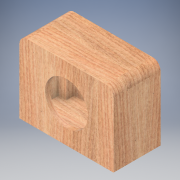
# Autodesk Inventor part: speakerBox
Saved by Autodesk Inventor 2017 (Build 210142000, 142)
## iProperties
Created: 2018-07-22
Part Number: speakerBox
Material: Wood (Birch)
Document SubType Name: Modeling
Designer: Jake
Density: 0.55 g/cm^3
Appearance: Birch - Natural Polished
Author: Jake
Autodesk Inventor part; units mm, degrees
ref_plane "YZ Plane" through (0, 0, 0) normal (1, 0, 0) x (0, 1, 0)
ref_plane "XZ Plane" through (0, 0, 0) normal (0, 1, 0) x (-1, 0, 0)
ref_plane "XY Plane" through (0, 0, 0) normal (0, 0, 1) x (1, 0, 0)
sketch "Sketch1" plane through (0, 0, 0) normal (0, 1, 0) x (-1, 0, 0)
  line L0 (152.4, 76.2) -> (-152.4, 76.2)
  line L1 (-152.4, 76.2) -> (-152.4, -76.2)
  line L2 (-152.4, -76.2) -> (152.4, -76.2)
  line L3 (152.4, -76.2) -> (152.4, 76.2)
  point P0 (0, 0)
  point P1 (152.4, 0)
  point P2 (0, -76.2)
  dimension "d0" = 152.4
  dimension "d1" = 304.8
  constraints: 8 end point, 2 midpoint, 2 parallel, 1 horizontal, 1 horizontal alignment, 1 perpendicular, 1 vertical alignment
  measures "d0" distance of L2.end L0.start
  measures "d1" distance of L1.end L2.end
extrude "Extrusion1" add sketch "Sketch1" along normal blind 15.875
sketch "Sketch4" plane through (0, 15.875, 0) normal (0, 1, 0) x (1, 0, 0)
  line L0 (-152.4, -76.2) -> (152.4, -76.2) projected
  line L1 (152.4, -76.2) -> (152.4, 76.2) projected
  line L2 (152.4, 76.2) -> (-152.4, 76.2) projected
  line L3 (-152.4, 76.2) -> (-152.4, -76.2) projected
  line L4 (-152.4, -76.2) -> (152.4, -76.2) projected
  line L5 (-152.4, -76.2) -> (136.525, -76.2)
  line L6 (136.525, -76.2) -> (136.525, -60.325)
  line L7 (136.525, -60.325) -> (-152.4, -60.325)
  line L8 (-152.4, -60.325) -> (-152.4, -76.2)
  point P0 (0, 0)
  dimension "d4" = 15.875
  dimension "d5" = 15.875
  constraints: 8 end point, 2 parallel, 1 horizontal, 1 perpendicular
  measures "d4" distance between parallel lines of L0 L7
  measures "d5" distance between parallel lines of L1 L6
extrude "Extrusion2" add sketch "Sketch4" along normal blind 203.2 contours L3 L7 L6 L0
sketch "Sketch5" plane through (0, 15.875, 0) normal (0, 1, 0) x (1, 0, 0)
  line L0 (136.525, -60.325) -> (136.525, -76.2) projected
  line L1 (136.525, -76.2) -> (152.4, -76.2) projected
  line L2 (152.4, -76.2) -> (152.4, 76.2) projected
  line L3 (152.4, 76.2) -> (-152.4, 76.2) projected
  line L4 (-152.4, 76.2) -> (-152.4, -60.325) projected
  line L5 (-152.4, -60.325) -> (136.525, -60.325) projected
  line L6 (-152.4, -76.2) -> (152.4, -76.2) projected
  line L7 (152.4, -76.2) -> (136.525, -76.2)
  line L8 (136.525, -76.2) -> (136.525, 60.325)
  line L9 (136.525, 60.325) -> (152.4, 60.325)
  line L10 (152.4, 60.325) -> (152.4, -76.2)
  line L11 (136.525, -76.2) -> (136.525, -60.325) projected
  point P0 (0, 0)
  dimension "d8" = 15.875
  constraints: 8 end point, 2 parallel, 1 collinear, 1 horizontal, 1 perpendicular
  measures "d8" distance between parallel lines of L3 L9
extrude "Extrusion3" add sketch "Sketch5" along normal blind 203.2 contours L8 L9 L2 L1 L0
sketch "Sketch6" plane through (0, 15.875, 0) normal (0, 1, 0) x (1, 0, 0)
  line L0 (136.525, 60.325) -> (152.4, 60.325) projected
  line L1 (152.4, 60.325) -> (152.4, 76.2) projected
  line L2 (152.4, 76.2) -> (-152.4, 76.2) projected
  line L3 (-152.4, 76.2) -> (-152.4, -60.325) projected
  line L4 (-152.4, -60.325) -> (136.525, -60.325) projected
  line L5 (136.525, -60.325) -> (136.525, 60.325) projected
  line L6 (152.4, 76.2) -> (-136.525, 76.2)
  line L7 (-136.525, 76.2) -> (-136.525, 60.325)
  line L8 (-136.525, 60.325) -> (152.4, 60.325)
  line L9 (152.4, 60.325) -> (152.4, 76.2)
  line L10 (152.4, 60.325) -> (136.525, 60.325) projected
  point P0 (0, 0)
  dimension "d11" = 15.875
  constraints: 8 end point, 2 parallel, 1 collinear, 1 horizontal, 1 perpendicular
  measures "d11" distance between parallel lines of L3 L7
extrude "Extrusion4" add sketch "Sketch6" along normal blind 203.2 contours L8 L7 L2 L1 L0
sketch "Sketch7" plane through (0, 15.875, 0) normal (0, 1, 0) x (1, 0, 0)
  line L0 (-136.525, 60.325) -> (-136.525, 76.2) projected
  line L1 (-136.525, 76.2) -> (-152.4, 76.2) projected
  line L2 (-152.4, 76.2) -> (-152.4, -60.325) projected
  line L3 (-152.4, -60.325) -> (136.525, -60.325) projected
  line L4 (136.525, -60.325) -> (136.525, 60.325) projected
  line L5 (136.525, 60.325) -> (-136.525, 60.325) projected
  line L6 (-152.4, -60.325) -> (136.525, -60.325) projected
  line L7 (-152.4, 76.2) -> (-136.525, 76.2)
  line L8 (-136.525, 76.2) -> (-136.525, -60.325)
  line L9 (-136.525, -60.325) -> (-152.4, -60.325)
  line L10 (-152.4, -60.325) -> (-152.4, 76.2)
  line L11 (-136.525, 76.2) -> (-136.525, 60.325) projected
  point P0 (0, 0)
  constraints: 8 end point, 2 parallel, 1 collinear, 1 horizontal, 1 perpendicular, 1 point on line
extrude "Extrusion5" add sketch "Sketch7" along normal blind 203.2 contours L8 L3 L2 L1 L0
sketch "Sketch8" plane through (0, 219.075, 0) normal (0, 1, 0) x (1, 0, 0)
  line L0 (136.525, -60.325) -> (-136.525, -60.325) projected
  line L1 (-152.4, 76.2) -> (-152.4, -76.2) projected
  line L2 (152.4, -76.2) -> (152.4, 76.2) projected
  line L3 (-152.4, 76.2) -> (152.4, 76.2)
  line L4 (152.4, 76.2) -> (152.4, -76.2)
  line L5 (152.4, -76.2) -> (-152.4, -76.2)
  line L6 (-152.4, -76.2) -> (-152.4, 76.2)
  line L7 (-152.4, -76.2) -> (152.4, -76.2) projected
  line L8 (136.525, 60.325) -> (136.525, -60.325) projected
  line L9 (152.4, -76.2) -> (152.4, 76.2) projected
  line L10 (-136.525, 60.325) -> (136.525, 60.325) projected
  line L11 (-136.525, -60.325) -> (-136.525, 60.325) projected
  line L12 (152.4, 76.2) -> (-152.4, 76.2) projected
  point P0 (0, 0)
  constraints: 8 end point, 2 collinear, 2 parallel, 1 horizontal, 1 perpendicular
extrude "Extrusion6" add sketch "Sketch8" along normal blind 15.875 contours L0 L11 L10 L8 | L3 L2 L5 L1
sketch "Sketch9" plane through (-152.4, 0, 76.2) normal (0, 0, 1) x (1, 0, 0)
  circle A0 centre (152.4, 117.475) radius 69.5
  line L0 (0, 0) -> (304.8, 0) projected
  line L1 (304.8, 0) -> (304.8, 234.95) projected
  line L2 (0, 0) -> (0, 234.95) projected
  line L3 (0, 234.95) -> (304.8, 234.95) projected
  line L4 (0, 234.95) -> (304.8, 234.95) projected
  point P0 (152.4, 0)
  point P1 (304.8, 117.475)
  point P2 (152.4, 234.95)
  point P3 (234.95, 190.5)
  point P4 (152.4, 234.95)
  dimension "d18" = 139
  constraints: 2 midpoint, 1 centre point, 1 horizontal alignment, 1 vertical alignment, 2 other
  measures "d18" diameter of A0
extrude "Extrusion7" cut sketch "Sketch9" against normal up to next contours A0
sketch "Sketch10" plane through (0, 15.875, 0) normal (0, 1, 0) x (1, 0, 0)
  line L0 (-136.525, 60.325) -> (-136.525, -60.325) projected
  line L1 (-136.525, -60.325) -> (136.525, -60.325) projected
  line L2 (136.525, -60.325) -> (136.525, 60.325) projected
  line L3 (136.525, 60.325) -> (-136.525, 60.325) projected
  line L4 (-136.525, 60.325) -> (-111.125, 60.325)
  line L5 (-111.125, 60.325) -> (-111.125, 34.925)
  line L6 (-111.125, 34.925) -> (-136.525, 34.925)
  line L7 (-136.525, 34.925) -> (-136.525, 60.325)
  line L8 (136.525, 60.325) -> (111.125, 60.325)
  line L9 (111.125, 60.325) -> (111.125, 34.925)
  line L10 (111.125, 34.925) -> (136.525, 34.925)
  line L11 (136.525, 34.925) -> (136.525, 60.325)
  line L12 (-136.525, -60.325) -> (-111.125, -60.325)
  line L13 (-111.125, -60.325) -> (-111.125, -34.925)
  line L14 (-111.125, -34.925) -> (-136.525, -34.925)
  line L15 (-136.525, -34.925) -> (-136.525, -60.325)
  line L16 (136.525, -60.325) -> (111.125, -60.325)
  line L17 (111.125, -60.325) -> (111.125, -34.925)
  line L18 (111.125, -34.925) -> (136.525, -34.925)
  line L19 (136.525, -34.925) -> (136.525, -60.325)
  point P0 (0, 0)
  dimension "d21" = 25.4
  dimension "d22" = 25.4
  dimension "d23" = 25.4
  dimension "d24" = 25.4
  dimension "d25" = 25.4
  dimension "d26" = 25.4
  constraints: 32 end point, 8 parallel, 4 horizontal, 4 perpendicular, 2 point on line
  measures "d21" distance of L4.end L5.end
  measures "d22" distance of L5.end L6.end
  measures "d23" distance of L9.end L10.end
  measures "d24" distance of L13.end L14.end
  measures "d25" distance of L12.end L13.end
  measures "d26" distance of L17.end L18.end
extrude "Extrusion8" add sketch "Sketch10" along normal up to surface (203.2 mm away) contours L3 L5 L6 L0 | L14 L13 L1 L0 | L3 L2 L10 L9 | L17 L18 L2 L1
fillet "Fillet1" radius 25.4 2 edges at (152.4, 234.95, 0) (-152.4, 234.95, 0)
equation "\"d5\" = d4"
body "Solid1"
